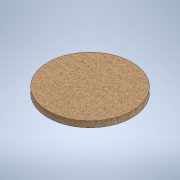
# Autodesk Inventor part: Soporte Eyección
Saved by Autodesk Inventor 2020 (Build 240168000, 168)
## iProperties
Created: 2021-10-18
Part Number: Soporte Eyección
Material: MDF Medium Density Fiberboard
Document SubType Name: Modeling
Designer: Carlos
Density: 0.8 g/cm^3
Appearance: Cardboard - Corrugated
Mass: 23.9314 g
Surface Area: 92.1272 cm^2
Volume: 29.9142 cm^3
Author: Carlos
Autodesk Inventor part; units mm, degrees
ref_plane "YZ Plane" through (0, 0, 0) normal (1, 0, 0) x (0, 1, 0)
ref_plane "XZ Plane" through (0, 0, 0) normal (0, 1, 0) x (-1, 0, 0)
ref_plane "XY Plane" through (0, 0, 0) normal (0, 0, 1) x (1, 0, 0)
sketch "Sketch1" plane through (0, 0, 0) normal (0, 1, 0) x (-1, 0, 0)
  circle A0 centre (0, 0) radius 34.5
  dimension "d0" = 69
  constraints: 1 centre point, 1 coincident
  measures "d0" diameter of A0
extrude "Extrusion1" add sketch "Sketch1" along normal mid plane 5
body "Solid1"
